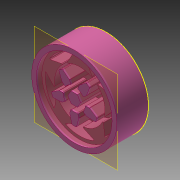
# Autodesk Inventor part: moldmaybe
Saved by Autodesk Inventor 2013 (Build 170138000, 138)
## iProperties
Created: 2013-05-10
Part Number: moldmaybe
Material: Rubber, Silicone
Document SubType Name: Modeling
Designer: grtstudent
Density: 1.25 g/cm^3
Mass: 147.324 g
Surface Area: 345.242 cm^2
Volume: 117.859 cm^3
Author: grtstudent
Autodesk Inventor part; units mm, degrees
ref_plane "YZ Plane" through (0, 0, 0) normal (1, 0, 0) x (0, 1, 0)
ref_plane "XZ Plane" through (0, 0, 0) normal (0, 1, 0) x (-1, 0, 0)
ref_plane "XY Plane" through (0, 0, 0) normal (0, 0, 1) x (1, 0, 0)
sketch "Sketch1" plane through (0, 0, 0) normal (0, 0, 1) x (1, 0, 0)
  circle A0 centre (0, 0) radius 42.8625
  dimension "d0" = 85.725
  constraints: 1 centre point, 1 coincident
  measures "d0" diameter of A0
extrude "Extrusion1" add sketch "Sketch1" along normal blind 31.75
sketch "Sketch2" plane through (0, 0, 31.75) normal (0, 0, 1) x (1, 0, 0)
  arc A0 (5.4223, 1.2129) -> (3.7615, 4.0894) centre (0, 0) ccw
  line L0 (5.4223, 1.2129) -> (6.1225, 0)
  line L1 (6.1225, 0) -> (5.4223, -1.2129)
  arc A1 (3.7615, -4.0894) -> (5.4223, -1.2129) centre (0, 0) ccw
  line L2 (3.7615, -4.0894) -> (3.0613, -5.3022)
  line L3 (3.0613, -5.3022) -> (1.6607, -5.3022)
  arc A2 (-1.6607, -5.3022) -> (1.6607, -5.3022) centre (0, 0) ccw
  line L4 (-1.6607, -5.3022) -> (-3.0613, -5.3022)
  line L5 (-3.0613, -5.3022) -> (-3.7615, -4.0894)
  arc A3 (-5.4223, -1.2129) -> (-3.7615, -4.0894) centre (0, 0) ccw
  line L6 (-5.4223, -1.2129) -> (-6.1225, 0)
  line L7 (-6.1225, 0) -> (-5.4223, 1.2129)
  arc A4 (-3.7615, 4.0894) -> (-5.4223, 1.2129) centre (0, 0) ccw
  line L8 (-3.7615, 4.0894) -> (-3.0613, 5.3022)
  line L9 (-3.0613, 5.3022) -> (-1.6607, 5.3022)
  arc A5 (1.6607, 5.3022) -> (-1.6607, 5.3022) centre (0, 0) ccw
  line L10 (1.6607, 5.3022) -> (3.0613, 5.3022)
  line L11 (3.0613, 5.3022) -> (3.7615, 4.0894)
  arc A6 (4.5235, -14.7334) -> (4.5231, -14.3404) centre (3.7871, -14.5376) ccw
  line L12 (4.5235, -14.7334) -> (2.3604, -22.8707)
  arc A7 (1.6784, -23.435) -> (2.3604, -22.8707) centre (1.6239, -22.6749) ccw
  arc A8 (-1.6784, -23.435) -> (1.6784, -23.435) centre (0, 0) ccw
  arc A9 (-2.3604, -22.8707) -> (-1.6784, -23.435) centre (-1.6239, -22.6749) ccw
  line L13 (-2.3604, -22.8707) -> (-4.5235, -14.7334)
  arc A10 (-4.5231, -14.3404) -> (-4.5235, -14.7334) centre (-3.7871, -14.5376) ccw
  line L14 (-4.5231, -14.3404) -> (-3.7082, -11.2993)
  arc A11 (-2.7815, -10.7588) -> (-3.7082, -11.2993) centre (-2.9722, -11.4965) ccw
  arc A12 (-2.7815, -10.7588) -> (2.7815, -10.7588) centre (0, 0) ccw
  arc A13 (3.7082, -11.2993) -> (2.7815, -10.7588) centre (2.9722, -11.4965) ccw
  line L15 (3.7082, -11.2993) -> (4.5231, -14.3404)
  arc A14 (15.4101, -0.2508) -> (15.0363, -0.1297) centre (14.9964, -0.8907) ccw
  line L16 (15.4101, -0.2508) -> (22.4807, -4.8226)
  arc A15 (22.8066, -5.6456) -> (22.4807, -4.8226) centre (22.067, -5.4625) ccw
  arc A16 (21.7693, -8.838) -> (22.8066, -5.6456) centre (0, 0) ccw
  arc A17 (21.0219, -9.3123) -> (21.7693, -8.838) centre (21.0633, -8.5514) ccw
  line L17 (21.0219, -9.3123) -> (12.6145, -8.855)
  arc A18 (12.2408, -8.7332) -> (12.6145, -8.855) centre (12.6559, -8.0941) ccw
  line L18 (12.2408, -8.7332) -> (9.6004, -7.0184)
  arc A19 (9.3727, -5.97) -> (9.6004, -7.0184) centre (10.0154, -6.3793) ccw
  arc A20 (9.3727, -5.97) -> (11.0917, -0.6793) centre (0, 0) ccw
  arc A21 (11.8922, 0.0351) -> (11.0917, -0.6793) centre (11.8523, -0.7259) ccw
  line L19 (11.8922, 0.0351) -> (15.0363, -0.1297)
  arc A22 (5.0005, 14.5784) -> (4.7698, 14.2603) centre (5.4812, 13.9872) ccw
  line L20 (5.0005, 14.5784) -> (11.5335, 19.8902)
  arc A23 (12.4169, 19.9458) -> (11.5335, 19.8902) centre (12.0142, 19.2989) ccw
  arc A24 (15.1326, 17.9728) -> (12.4169, 19.9458) centre (0, 0) ccw
  arc A25 (15.3526, 17.1154) -> (15.1326, 17.9728) centre (14.6418, 17.3899) ccw
  line L21 (15.3526, 17.1154) -> (12.3197, 9.2607)
  arc A26 (12.0883, 8.943) -> (12.3197, 9.2607) centre (11.6088, 9.5352) ccw
  line L22 (12.0883, 8.943) -> (9.6416, 6.9617)
  arc A27 (8.5741, 7.0691) -> (9.6416, 6.9617) centre (9.162, 7.5539) ccw
  arc A28 (8.5741, 7.0691) -> (4.0736, 10.3389) centre (0, 0) ccw
  arc A29 (3.6415, 11.321) -> (4.0736, 10.3389) centre (4.3529, 11.0479) ccw
  line L23 (3.6415, 11.321) -> (4.7698, 14.2603)
  arc A30 (-12.3197, 9.2607) -> (-12.0883, 8.943) centre (-11.6088, 9.5352) ccw
  line L24 (-12.3197, 9.2607) -> (-15.3526, 17.1154)
  arc A31 (-15.1326, 17.9728) -> (-15.3526, 17.1154) centre (-14.6418, 17.3899) ccw
  arc A32 (-12.4169, 19.9458) -> (-15.1326, 17.9728) centre (0, 0) ccw
  arc A33 (-11.5335, 19.8902) -> (-12.4169, 19.9458) centre (-12.0142, 19.2989) ccw
  line L25 (-11.5335, 19.8902) -> (-5.0005, 14.5784)
  arc A34 (-4.7698, 14.2603) -> (-5.0005, 14.5784) centre (-5.4812, 13.9872) ccw
  line L26 (-4.7698, 14.2603) -> (-3.6415, 11.321)
  arc A35 (-4.0736, 10.3389) -> (-3.6415, 11.321) centre (-4.3529, 11.0479) ccw
  arc A36 (-4.0736, 10.3389) -> (-8.5741, 7.0691) centre (0, 0) ccw
  arc A37 (-9.6416, 6.9617) -> (-8.5741, 7.0691) centre (-9.162, 7.5539) ccw
  line L27 (-9.6416, 6.9617) -> (-12.0883, 8.943)
  arc A38 (-12.6145, -8.855) -> (-12.2408, -8.7332) centre (-12.6559, -8.0941) ccw
  line L28 (-12.6145, -8.855) -> (-21.0219, -9.3123)
  arc A39 (-21.7693, -8.838) -> (-21.0219, -9.3123) centre (-21.0633, -8.5514) ccw
  arc A40 (-22.8066, -5.6456) -> (-21.7693, -8.838) centre (0, 0) ccw
  arc A41 (-22.4807, -4.8226) -> (-22.8066, -5.6456) centre (-22.067, -5.4625) ccw
  line L29 (-22.4807, -4.8226) -> (-15.4101, -0.2508)
  arc A42 (-15.0363, -0.1297) -> (-15.4101, -0.2508) centre (-14.9964, -0.8907) ccw
  line L30 (-15.0363, -0.1297) -> (-11.8922, 0.0351)
  arc A43 (-11.0917, -0.6793) -> (-11.8922, 0.0351) centre (-11.8523, -0.7259) ccw
  arc A44 (-11.0917, -0.6793) -> (-9.3727, -5.97) centre (0, 0) ccw
  arc A45 (-9.6004, -7.0184) -> (-9.3727, -5.97) centre (-10.0154, -6.3793) ccw
  line L31 (-9.6004, -7.0184) -> (-12.2408, -8.7332)
  circle A46 centre (-18.1176, 5.8868) radius 1.905
  circle A47 centre (11.1973, -15.4118) radius 1.905
  circle A48 centre (0, 19.05) radius 1.905
  circle A49 centre (18.1176, 5.8868) radius 1.905
  circle A50 centre (-11.1973, -15.4118) radius 1.905
  circle A51 centre (0, 0) radius 38.1
  constraints: 92 point on circle, 64 end point, 52 centre point
extrude "Extrusion2" cut sketch "Sketch2" against normal blind 23.8125
sketch "Sketch3" plane through (0, 0, 7.9375) normal (0, 0, 1) x (1, 0, 0)
  line L0 (12.2408, -8.7332) -> (9.6004, -7.0184)
  arc A0 (9.3727, -5.97) -> (9.6004, -7.0184) centre (10.0154, -6.3793) ccw
  arc A1 (9.3727, -5.97) -> (11.0917, -0.6793) centre (0, 0) ccw
  arc A2 (11.8922, 0.0351) -> (11.0917, -0.6793) centre (11.8523, -0.7259) ccw
  line L1 (11.8922, 0.0351) -> (15.0363, -0.1297)
  arc A3 (15.4101, -0.2508) -> (15.0363, -0.1297) centre (14.9964, -0.8907) ccw
  line L2 (15.4101, -0.2508) -> (22.4807, -4.8226)
  arc A4 (22.8066, -5.6456) -> (22.4807, -4.8226) centre (22.067, -5.4625) ccw
  arc A5 (21.7693, -8.838) -> (22.8066, -5.6456) centre (0, 0) ccw
  arc A6 (21.0219, -9.3123) -> (21.7693, -8.838) centre (21.0633, -8.5514) ccw
  line L3 (21.0219, -9.3123) -> (12.6145, -8.855)
  arc A7 (12.2408, -8.7332) -> (12.6145, -8.855) centre (12.6559, -8.0941) ccw
  line L4 (12.0883, 8.943) -> (9.6416, 6.9617)
  arc A8 (8.5741, 7.0691) -> (9.6416, 6.9617) centre (9.162, 7.5539) ccw
  arc A9 (8.5741, 7.0691) -> (4.0736, 10.3389) centre (0, 0) ccw
  arc A10 (3.6415, 11.321) -> (4.0736, 10.3389) centre (4.3529, 11.0479) ccw
  line L5 (3.6415, 11.321) -> (4.7698, 14.2603)
  arc A11 (5.0005, 14.5784) -> (4.7698, 14.2603) centre (5.4812, 13.9872) ccw
  line L6 (5.0005, 14.5784) -> (11.5335, 19.8902)
  arc A12 (12.4169, 19.9458) -> (11.5335, 19.8902) centre (12.0142, 19.2989) ccw
  arc A13 (15.1326, 17.9728) -> (12.4169, 19.9458) centre (0, 0) ccw
  arc A14 (15.3526, 17.1154) -> (15.1326, 17.9728) centre (14.6418, 17.3899) ccw
  line L7 (15.3526, 17.1154) -> (12.3197, 9.2607)
  arc A15 (12.0883, 8.943) -> (12.3197, 9.2607) centre (11.6088, 9.5352) ccw
  line L8 (-4.7698, 14.2603) -> (-3.6415, 11.321)
  arc A16 (-4.0736, 10.3389) -> (-3.6415, 11.321) centre (-4.3529, 11.0479) ccw
  arc A17 (-4.0736, 10.3389) -> (-8.5741, 7.0691) centre (0, 0) ccw
  arc A18 (-9.6416, 6.9617) -> (-8.5741, 7.0691) centre (-9.162, 7.5539) ccw
  line L9 (-9.6416, 6.9617) -> (-12.0883, 8.943)
  arc A19 (-12.3197, 9.2607) -> (-12.0883, 8.943) centre (-11.6088, 9.5352) ccw
  line L10 (-12.3197, 9.2607) -> (-15.3526, 17.1154)
  arc A20 (-15.1326, 17.9728) -> (-15.3526, 17.1154) centre (-14.6418, 17.3899) ccw
  arc A21 (-12.4169, 19.9458) -> (-15.1326, 17.9728) centre (0, 0) ccw
  arc A22 (-11.5335, 19.8902) -> (-12.4169, 19.9458) centre (-12.0142, 19.2989) ccw
  line L11 (-11.5335, 19.8902) -> (-5.0005, 14.5784)
  arc A23 (-4.7698, 14.2603) -> (-5.0005, 14.5784) centre (-5.4812, 13.9872) ccw
  line L12 (-15.0363, -0.1297) -> (-11.8922, 0.0351)
  arc A24 (-11.0917, -0.6793) -> (-11.8922, 0.0351) centre (-11.8523, -0.7259) ccw
  arc A25 (-11.0917, -0.6793) -> (-9.3727, -5.97) centre (0, 0) ccw
  arc A26 (-9.6004, -7.0184) -> (-9.3727, -5.97) centre (-10.0154, -6.3793) ccw
  line L13 (-9.6004, -7.0184) -> (-12.2408, -8.7332)
  arc A27 (-12.6145, -8.855) -> (-12.2408, -8.7332) centre (-12.6559, -8.0941) ccw
  line L14 (-12.6145, -8.855) -> (-21.0219, -9.3123)
  arc A28 (-21.7693, -8.838) -> (-21.0219, -9.3123) centre (-21.0633, -8.5514) ccw
  arc A29 (-22.8066, -5.6456) -> (-21.7693, -8.838) centre (0, 0) ccw
  arc A30 (-22.4807, -4.8226) -> (-22.8066, -5.6456) centre (-22.067, -5.4625) ccw
  line L15 (-22.4807, -4.8226) -> (-15.4101, -0.2508)
  arc A31 (-15.0363, -0.1297) -> (-15.4101, -0.2508) centre (-14.9964, -0.8907) ccw
  line L16 (-4.5231, -14.3404) -> (-3.7082, -11.2993)
  arc A32 (-2.7815, -10.7588) -> (-3.7082, -11.2993) centre (-2.9722, -11.4965) ccw
  arc A33 (-2.7815, -10.7588) -> (2.7815, -10.7588) centre (0, 0) ccw
  arc A34 (3.7082, -11.2993) -> (2.7815, -10.7588) centre (2.9722, -11.4965) ccw
  line L17 (3.7082, -11.2993) -> (4.5231, -14.3404)
  arc A35 (4.5235, -14.7334) -> (4.5231, -14.3404) centre (3.7871, -14.5376) ccw
  line L18 (4.5235, -14.7334) -> (2.3604, -22.8707)
  arc A36 (1.6784, -23.435) -> (2.3604, -22.8707) centre (1.6239, -22.6749) ccw
  arc A37 (-1.6784, -23.435) -> (1.6784, -23.435) centre (0, 0) ccw
  arc A38 (-2.3604, -22.8707) -> (-1.6784, -23.435) centre (-1.6239, -22.6749) ccw
  line L19 (-2.3604, -22.8707) -> (-4.5235, -14.7334)
  arc A39 (-4.5231, -14.3404) -> (-4.5235, -14.7334) centre (-3.7871, -14.5376) ccw
  circle A40 centre (11.1973, -15.4118) radius 1.905
  circle A41 centre (-18.1176, 5.8868) radius 1.905
  circle A42 centre (0, 19.05) radius 1.905
  circle A43 centre (-11.1973, -15.4118) radius 1.905
  circle A44 centre (18.1176, 5.8868) radius 1.905
  line L20 (-3.2079, 5.5562) -> (3.2079, 5.5562)
  line L21 (3.2079, 5.5562) -> (6.4158, 0)
  line L22 (6.4158, 0) -> (3.2079, -5.5562)
  line L23 (3.2079, -5.5562) -> (-3.2079, -5.5562)
  line L24 (-3.2079, -5.5562) -> (-6.4158, 0)
  line L25 (-6.4158, 0) -> (-3.2079, 5.5562)
  arc A45 (13.8588, -32.0576) -> (13.873, -30.9711) centre (13.6226, -31.5111) ccw
  line L26 (13.873, -30.9711) -> (3.6675, -26.2384)
  arc A46 (3.8282, -25.1098) -> (3.6675, -26.2384) centre (3.918, -25.6984) ccw
  arc A47 (3.8282, -25.1098) -> (22.6979, -11.4002) centre (0, 0) ccw
  arc A48 (23.8209, -11.5961) -> (22.6979, -11.4002) centre (23.2299, -11.6674) ccw
  line L27 (23.8209, -11.5961) -> (25.1682, -22.7646)
  arc A49 (25.1682, -22.7646) -> (26.206, -23.0869) centre (25.7593, -22.6933) ccw
  arc A50 (26.206, -23.0869) -> (34.7712, 3.2742) centre (0, 0) ccw
  arc A51 (34.7712, 3.2742) -> (33.7423, 3.6235) centre (34.1785, 3.2184) ccw
  line L28 (33.7423, 3.6235) -> (26.0876, -4.6201)
  arc A52 (25.0639, -4.1185) -> (26.0876, -4.6201) centre (25.6513, -4.215) ccw
  arc A53 (25.0639, -4.1185) -> (17.8563, 18.0641) centre (0, 0) ccw
  arc A54 (18.3896, 19.0716) -> (17.8563, 18.0641) centre (18.2748, 18.4875) ccw
  line L29 (18.3896, 19.0716) -> (29.4279, 16.9018)
  arc A55 (29.4279, 16.9018) -> (30.055, 17.7891) centre (29.5427, 17.4859) ccw
  arc A56 (30.055, 17.7891) -> (7.631, 34.0811) centre (0, 0) ccw
  arc A57 (7.631, 34.0811) -> (6.9808, 33.2105) centre (7.5009, 33.5002) ccw
  line L30 (6.9808, 33.2105) -> (12.4555, 23.383)
  arc A58 (11.6621, 22.5645) -> (12.4555, 23.383) centre (11.9354, 23.0933) ccw
  arc A59 (11.6621, 22.5645) -> (-11.6621, 22.5645) centre (0, 0) ccw
  arc A60 (-12.4555, 23.383) -> (-11.6621, 22.5645) centre (-11.9354, 23.0933) ccw
  line L31 (-12.4555, 23.383) -> (-6.9808, 33.2105)
  arc A61 (-6.9808, 33.2105) -> (-7.631, 34.0811) centre (-7.5009, 33.5002) ccw
  arc A62 (-7.631, 34.0811) -> (-30.055, 17.7891) centre (0, 0) ccw
  arc A63 (-30.055, 17.7891) -> (-29.4279, 16.9018) centre (-29.5427, 17.4859) ccw
  line L32 (-29.4279, 16.9018) -> (-18.3896, 19.0716)
  arc A64 (-17.8563, 18.0641) -> (-18.3896, 19.0716) centre (-18.2748, 18.4875) ccw
  arc A65 (-17.8563, 18.0641) -> (-25.0639, -4.1185) centre (0, 0) ccw
  arc A66 (-26.0876, -4.6201) -> (-25.0639, -4.1185) centre (-25.6513, -4.215) ccw
  line L33 (-26.0876, -4.6201) -> (-33.7423, 3.6235)
  arc A67 (-33.7423, 3.6235) -> (-34.7712, 3.2742) centre (-34.1785, 3.2184) ccw
  arc A68 (-34.7712, 3.2742) -> (-26.206, -23.0869) centre (0, 0) ccw
  arc A69 (-26.206, -23.0869) -> (-25.1682, -22.7646) centre (-25.7593, -22.6933) ccw
  line L34 (-25.1682, -22.7646) -> (-23.8209, -11.5961)
  arc A70 (-22.6979, -11.4002) -> (-23.8209, -11.5961) centre (-23.2299, -11.6674) ccw
  arc A71 (-22.6979, -11.4002) -> (-3.8282, -25.1098) centre (0, 0) ccw
  arc A72 (-3.6675, -26.2384) -> (-3.8282, -25.1098) centre (-3.918, -25.6984) ccw
  line L35 (-3.6675, -26.2384) -> (-13.873, -30.9711)
  arc A73 (-13.873, -30.9711) -> (-13.8588, -32.0576) centre (-13.6226, -31.5111) ccw
  arc A74 (-13.8588, -32.0576) -> (13.8588, -32.0576) centre (0, 0) ccw
  circle A75 centre (0, 0) radius 38.1 projected
  constraints: 140 point on circle, 75 centre point, 72 end point
extrude "Extrusion3" add sketch "Sketch3" along normal blind 18.2563 contours A75
sketch "Sketch4" plane through (11.1973, -15.4118, 31.75) normal (0, 0, 1) x (1, 0, 0)
  circle A0 centre (-11.1973, 34.4618) radius 1.905 projected
  circle A1 centre (-29.3149, 21.2985) radius 1.905 projected
  circle A2 centre (-22.3946, 0) radius 1.905 projected
  circle A3 centre (0, 0) radius 1.905 projected
  circle A4 centre (6.9203, 21.2985) radius 1.905 projected
  point P0 (-11.1973, 15.4118)
extrude "Extrusion4" cut sketch "Sketch4" against normal through all
sketch "Sketch5" plane through (0, 0, 31.75) normal (0, 0, 1) x (1, 0, 0)
  line L0 (-3.2079, 5.5563) -> (3.2079, 5.5563)
  line L1 (3.2079, 5.5563) -> (6.4158, 0)
  line L2 (6.4158, 0) -> (3.2079, -5.5562)
  line L3 (3.2079, -5.5562) -> (-3.2079, -5.5562)
  line L4 (-3.2079, -5.5562) -> (-6.4158, 0)
  line L5 (-6.4158, 0) -> (-3.2079, 5.5563)
  line L6 (-1.6607, 5.3022) -> (-3.0613, 5.3022) projected
  line L7 (3.0613, 5.3022) -> (1.6607, 5.3022) projected
  arc A0 (1.6607, 5.3022) -> (-1.6607, 5.3022) centre (0, 0) ccw projected
  constraints: 12 end point, 1 coincident, 1 parallel, 1 tangent, 13 other
extrude "Extrusion5" add sketch "Sketch5" against normal up to surface (23.8125 mm away)
ref_plane "Work Plane1" through (0, 0, 30.1625) normal (0, 0, 1) x (1, 0, 0)
sketch "Sketch6" plane through (0, 0, 0) normal (0, 0, -1) x (-1, 0, 0)
  circle A0 centre (-11.1973, -15.4118) radius 1.905 projected
  circle A1 centre (18.1176, 5.8868) radius 1.905 projected
  circle A2 centre (0, 19.05) radius 1.905 projected
  circle A3 centre (11.1973, -15.4118) radius 1.905 projected
  circle A4 centre (-18.1176, 5.8868) radius 1.905 projected
  circle A5 centre (0, 0) radius 42.8625 projected
body "Solid1"
